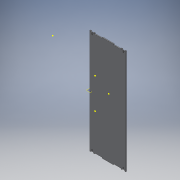
# Autodesk Inventor part: ProjectorMount 1
Saved by Autodesk Inventor 2019 (Build 230136000, 136)
## iProperties
Created: 2020-03-21
Part Number: ProjectorMount 1
Material: Generic
Document SubType Name: Modeling
Designer: Vijay
Density: 1 g/cm^3
Appearance: Default
Author: Vijay
Autodesk Inventor part; units mm, degrees
ref_plane "YZ Plane" through (0, 0, 0) normal (1, 0, 0) x (0, 1, 0)
ref_plane "XZ Plane" through (0, 0, 0) normal (0, 1, 0) x (-1, 0, 0)
ref_plane "XY Plane" through (0, 0, 0) normal (0, 0, 1) x (1, 0, 0)
sketch "Sketch2" plane through (0, 0, 0) normal (0, 0, 1) x (1, 0, 0)
  line L0 (204.4388, 124.4349) -> (404.4388, 124.4349)
  line L1 (404.4388, 124.4349) -> (404.4388, -445.5651)
  line L2 (404.4388, -445.5651) -> (204.4388, -445.5651)
  line L3 (204.4388, -445.5651) -> (204.4388, 124.4349)
  point P0 (0, 0)
  point P1 (1605.8001, 124.4349)
  point P2 (1605.8004, -445.5651)
  dimension "d0" = 200
  constraints: 8 end point, 2 parallel, 2 point on line, 1 horizontal, 1 perpendicular, 2 other
  measures "d0" distance of L0.start L0.end
extrude "Extrusion1" add sketch "Sketch2" along normal blind 4
sketch "Sketch3" plane through (0, 0, 4) normal (0, 0, 1) x (1, 0, 0)
  arc A0 (204.9388, 128.7849) -> (204.4388, 128.2849) centre (204.9388, 128.2849) ccw projected
  line L0 (204.4388, 124.4349) -> (204.4388, 128.2849) projected
  line L1 (197.563, 124.4349) -> (204.4388, 124.4349) projected
  line L2 (197.563, 109.7813) -> (197.563, 124.4349) projected
  line L3 (238.5147, 109.7813) -> (197.563, 109.7813) projected
  line L4 (238.5147, 124.4349) -> (238.5147, 109.7813) projected
  line L5 (231.6388, 124.4349) -> (238.5147, 124.4349) projected
  line L6 (231.6388, 128.2849) -> (231.6388, 124.4349) projected
  arc A1 (231.6388, 128.2849) -> (231.1388, 128.7849) centre (231.1388, 128.2849) ccw projected
  line L7 (231.1388, 128.7849) -> (226.1388, 128.7849) projected
  arc A2 (226.1388, 128.7849) -> (225.6388, 128.2849) centre (226.1388, 128.2849) ccw projected
  line L8 (225.6388, 124.4349) -> (225.6388, 128.2849) projected
  line L9 (219.7388, 124.4349) -> (225.6388, 124.4349) projected
  line L10 (219.7388, 124.4349) -> (219.7388, 118.6349) projected
  line L11 (219.7388, 118.6349) -> (220.9888, 118.6349) projected
  line L12 (220.9888, 118.6349) -> (220.9888, 116.2349) projected
  line L13 (220.9888, 116.2349) -> (219.7388, 116.2349) projected
  line L14 (219.7388, 116.2349) -> (219.7388, 113.5849) projected
  line L15 (219.7388, 113.5849) -> (216.3388, 113.5849) projected
  line L16 (216.3388, 113.5849) -> (216.3388, 116.2349) projected
  line L17 (216.3388, 116.2349) -> (215.0888, 116.2349) projected
  line L18 (215.0888, 116.2349) -> (215.0888, 118.6349) projected
  line L19 (215.0888, 118.6349) -> (216.3388, 118.6349) projected
  line L20 (216.3388, 118.6349) -> (216.3388, 124.4349) projected
  line L21 (210.4388, 124.4349) -> (216.3388, 124.4349) projected
  line L22 (210.4388, 128.2849) -> (210.4388, 124.4349) projected
  arc A3 (210.4388, 128.2849) -> (209.9388, 128.7849) centre (209.9388, 128.2849) ccw projected
  line L23 (209.9388, 128.7849) -> (204.9388, 128.7849) projected
  arc A4 (377.7388, 128.7849) -> (377.2388, 128.2849) centre (377.7388, 128.2849) ccw projected
  line L24 (377.2388, 124.4349) -> (377.2388, 128.2849) projected
  line L25 (370.363, 124.4349) -> (377.2388, 124.4349) projected
  line L26 (370.363, 109.7813) -> (370.363, 124.4349) projected
  line L27 (411.3147, 109.7813) -> (370.363, 109.7813) projected
  line L28 (411.3147, 124.4349) -> (411.3147, 109.7813) projected
  line L29 (404.4388, 124.4349) -> (411.3147, 124.4349) projected
  line L30 (404.4388, 128.2849) -> (404.4388, 124.4349) projected
  arc A5 (404.4388, 128.2849) -> (403.9388, 128.7849) centre (403.9388, 128.2849) ccw projected
  line L31 (403.9388, 128.7849) -> (398.9388, 128.7849) projected
  arc A6 (398.9388, 128.7849) -> (398.4388, 128.2849) centre (398.9388, 128.2849) ccw projected
  line L32 (398.4388, 124.4349) -> (398.4388, 128.2849) projected
  line L33 (392.5388, 124.4349) -> (398.4388, 124.4349) projected
  line L34 (392.5388, 124.4349) -> (392.5388, 118.6349) projected
  line L35 (392.5388, 118.6349) -> (393.7888, 118.6349) projected
  line L36 (393.7888, 118.6349) -> (393.7888, 116.2349) projected
  line L37 (393.7888, 116.2349) -> (392.5388, 116.2349) projected
  line L38 (392.5388, 116.2349) -> (392.5388, 113.5849) projected
  line L39 (392.5388, 113.5849) -> (389.1388, 113.5849) projected
  line L40 (389.1388, 113.5849) -> (389.1388, 116.2349) projected
  line L41 (389.1388, 116.2349) -> (387.8888, 116.2349) projected
  line L42 (387.8888, 116.2349) -> (387.8888, 118.6349) projected
  line L43 (387.8888, 118.6349) -> (389.1388, 118.6349) projected
  line L44 (389.1388, 118.6349) -> (389.1388, 124.4349) projected
  line L45 (383.2388, 124.4349) -> (389.1388, 124.4349) projected
  line L46 (383.2388, 128.2849) -> (383.2388, 124.4349) projected
  arc A7 (383.2388, 128.2849) -> (382.7388, 128.7849) centre (382.7388, 128.2849) ccw projected
  line L47 (382.7388, 128.7849) -> (377.7388, 128.7849) projected
  line L48 (216.3388, 124.4349) -> (219.7388, 124.4349)
  line L49 (404.4388, 124.4349) -> (204.4388, 124.4349) projected
  line L50 (389.1388, 124.4349) -> (392.5388, 124.4349)
  point P0 (0, 0)
  constraints: 4 end point, 1 horizontal, 1 parallel, 1 other
extrude "Extrusion2" cut sketch "Sketch3" against normal blind 4 contours L48 L10 L11 L12 L13 L14 L15 L16 L17 L18 L19 L20 | L49 L34 L35 L36 L37 L38 L39 L40 L41 L42 L43 L44
sketch "Sketch5" plane through (0, 0, 0) normal (0, 0, -1) x (-1, 0, 0)
  line L0 (-210.4388, 124.4349) -> (-204.4388, 124.4349) projected
  line L1 (-204.4388, 128.2849) -> (-204.4388, 124.4349) projected
  arc A0 (-204.4388, 128.2849) -> (-204.9388, 128.7849) centre (-204.9388, 128.2849) ccw projected
  line L2 (-209.9388, 128.7849) -> (-204.9388, 128.7849) projected
  arc A1 (-209.9388, 128.7849) -> (-210.4388, 128.2849) centre (-209.9388, 128.2849) ccw projected
  line L3 (-210.4388, 124.4349) -> (-210.4388, 128.2849) projected
  line L4 (-231.6388, 124.4349) -> (-225.6388, 124.4349) projected
  line L5 (-225.6388, 128.2849) -> (-225.6388, 124.4349) projected
  arc A2 (-225.6388, 128.2849) -> (-226.1388, 128.7849) centre (-226.1388, 128.2849) ccw projected
  line L6 (-231.1388, 128.7849) -> (-226.1388, 128.7849) projected
  arc A3 (-231.1388, 128.7849) -> (-231.6388, 128.2849) centre (-231.1388, 128.2849) ccw projected
  line L7 (-231.6388, 124.4349) -> (-231.6388, 128.2849) projected
  line L8 (-383.2388, 124.4349) -> (-377.2388, 124.4349) projected
  line L9 (-377.2388, 128.2849) -> (-377.2388, 124.4349) projected
  arc A4 (-377.2388, 128.2849) -> (-377.7388, 128.7849) centre (-377.7388, 128.2849) ccw projected
  line L10 (-382.7388, 128.7849) -> (-377.7388, 128.7849) projected
  arc A5 (-382.7388, 128.7849) -> (-383.2388, 128.2849) centre (-382.7388, 128.2849) ccw projected
  line L11 (-383.2388, 124.4349) -> (-383.2388, 128.2849) projected
  line L12 (-404.4388, 124.4349) -> (-398.4388, 124.4349) projected
  line L13 (-398.4388, 128.2849) -> (-398.4388, 124.4349) projected
  arc A6 (-398.4388, 128.2849) -> (-398.9388, 128.7849) centre (-398.9388, 128.2849) ccw projected
  line L14 (-403.9388, 128.7849) -> (-398.9388, 128.7849) projected
  arc A7 (-403.9388, 128.7849) -> (-404.4388, 128.2849) centre (-403.9388, 128.2849) ccw projected
  line L15 (-404.4388, 124.4349) -> (-404.4388, 128.2849) projected
  point P0 (0, 0)
extrude "Extrusion4" add sketch "Sketch5" against normal blind 4
sketch "Sketch6" plane through (0, 0, 0) normal (0, 0, -1) x (-1, 0, 0)
  line L0 (-216.3388, 124.4349) -> (-216.3388, 118.6349) construction
  line L1 (-219.7388, 118.6349) -> (-219.7388, 124.4349) construction
  line L2 (-216.3388, 123.5848) -> (-219.7388, 123.5848)
  line L3 (-219.7388, 123.5848) -> (-219.7388, 126.4497)
  line L4 (-219.7388, 126.4497) -> (-216.3388, 126.4497)
  line L5 (-216.3388, 126.4497) -> (-216.3388, 123.5848)
  point P0 (0, 0)
  constraints: 8 end point, 2 parallel, 1 horizontal, 1 perpendicular, 1 point on line
extrude "Extrusion5" cut sketch "Sketch6" against normal through all
ref_plane "Work Plane1" through (204.4388, -160.5651, 0) normal (0, -1, 0) x (1, 0, 0)
mirror "Mirror1" about plane through (204.4388, -160.5651, 0) normal (0, -1, 0) of "Extrusion4", "Extrusion2"
sketch "Sketch7" plane through (0, 0, 4) normal (0, 0, 1) x (1, 0, 0)
  circle A0 centre (234.4388, -243.0651) radius 2 projected
  circle A1 centre (234.4388, -73.0651) radius 2 projected
  circle A2 centre (309.4388, -123.0651) radius 2 projected
  point P0 (0, 0)
sketch "Sketch8" plane through (0, 0, 4) normal (0, 0, 1) x (1, 0, 0)
  line L0 (204.4388, 124.4349) -> (204.4388, -445.5651) construction
  line L1 (196.4388, -445.5651) -> (553.2389, -445.5651) projected
  line L2 (377.2388, -445.5651) -> (231.6388, -445.5651) construction
  line L3 (304.4388, -445.5651) -> (304.4388, 124.4349) construction
  line L4 (377.2388, 124.4349) -> (231.6388, 124.4349) construction
  line L5 (336.1888, 128.7849) -> (336.1888, -449.9151)
  line L6 (336.1888, -449.9151) -> (272.6888, -449.9151)
  line L7 (272.6888, -449.9151) -> (272.6888, 128.7849)
  line L8 (272.6888, 128.7849) -> (336.1888, 128.7849)
  line L9 (336.1888, 128.7849) -> (272.6888, -449.9151) construction
  line L10 (336.1888, -449.9151) -> (272.6888, 128.7849) construction
  line L11 (231.1388, -449.9151) -> (226.1388, -449.9151) projected
  point P0 (0, 0)
  point P1 (304.4388, -160.5651)
  dimension "d11" = 63.5
  constraints: 14 end point, 5 midpoint, 2 parallel, 1 collinear, 1 perpendicular
  measures "d11" distance of L5.end L6.end
extrude "Extrusion6" add sketch "Sketch8" against normal blind 4
fillet "Fillet1" radius 1 4 edges at (272.6888, -449.9151, 2) (336.1888, -449.9151, 2) (272.6888, 128.7849, 2) (336.1888, 128.7849, 2)
sketch "Sketch9" plane through (0, 0, 4) normal (0, 0, 1) x (1, 0, 0)
  circle A0 centre (49.4388, -138.0651) radius 2 projected
  circle A1 centre (109.4388, -138.0651) radius 2 projected
  arc A2 (36.9461, -122.4468) -> (40.1047, -155.7533) centre (49.4388, -138.0651) ccw
  line L0 (36.9461, -122.4468) -> (204.4388, 11.5276)
  line L1 (204.4388, -445.5651) -> (204.4388, 124.4349) projected
  line L2 (40.1047, -155.7533) -> (204.4388, -242.4724)
  point P0 (0, 0)
  dimension "d15" = 40
  dimension "d16" = 254
  constraints: 4 end point, 2 point on circle, 2 point on line, 2 tangent, 1 centre point, 1 coincident
  measures "d15" diameter of A2
  measures "d16" distance of L0.end L2.end
extrude "Extrusion7" add sketch "Sketch9" against normal blind 4
fillet "Fillet2" radius 20 2 edges at (204.4388, 11.5276, 2) (204.4388, -242.4724, 2)
extrude "Extrusion8" cut sketch "Sketch7" against normal blind 4
body "Solid1"
